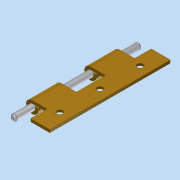
# Autodesk Inventor part: DIV
Saved by Autodesk Inventor 2012 SP1 (Build 160190100, 190)
## iProperties
Created: 2014-07-01
Material: Ms58
Document SubType Name: Modeling
Designer: Eisele
Density: 8.47 g/cm^3
Description: Schanier
Mass: 17.612 g
Surface Area: 32.73 cm^2
Volume: 2.07934 cm^3
Benennung: Schanier
Unterbennenung: 30x26x0,9
Projekt: DIV
Unterprojekt: Schanier
Author: Eisele
Title: DIV
Autodesk Inventor part; units mm, degrees
ref_plane "YZ Plane" through (0, 0, 0) normal (1, 0, 0) x (0, 1, 0)
ref_plane "XZ Plane" through (0, 0, 0) normal (0, 1, 0) x (-1, 0, 0)
ref_plane "XY Plane" through (0, 0, 0) normal (0, 0, 1) x (1, 0, 0)
sketch "Skizze1" plane through (0, 0, 0) normal (0, 1, 0) x (-1, 0, 0)
  line L0 (0, 0) -> (0, 79.9753) construction
  line L1 (0, 0) -> (-80.4332, 0) construction
  line L2 (0, 0) -> (80.1339, 0) construction
  line L3 (0, 0) -> (0, -79.3949) construction
  line L4 (0, 1.55) -> (-17, 1.55)
  line L5 (-17, 1.55) -> (-17, 2.95)
  line L6 (-17, 2.95) -> (0, 2.95)
  arc A0 (-1.3565, 0.75) -> (0, 1.55) centre (0, 0) ccw
  arc A1 (-2.8531, 0.75) -> (0, 2.95) centre (0, 0) ccw
  line L7 (-1.3565, 0.75) -> (-2.8531, 0.75)
  circle A2 centre (0, 0) radius 1.5
  dimension "d0" = 1.4
  dimension "d1" = 5.9
  dimension "d2" = 0.8
  dimension "d3" = 19.95
  dimension "d21" = 0.05
  dimension "d27" = 17
  constraints: 16 end point, 4 perpendicular, 4 point on circle, 3 centre point, 3 coincident, 2 parallel, 2 tangent, 1 collinear, 1 vertical
  measures "d0" distance between parallel lines of L6 L4
  measures "d1" diameter of A1
  measures "d2" distance between parallel lines of L4 L7
  measures "d21" radial gap between concentric circles of A0 A2
  measures "d27" distance from line of L4.end L3
extrude "Extrusion1" add sketch "Skizze1" along normal mid plane 60 contours L4 L5 L6 A1 L7 A0
sketch "Skizze3" plane through (0, 0, 0) normal (0, 0, 1) x (1, 0, 0)
  line L0 (5, -7.25) -> (-9.5, -7.25)
  line L1 (-9.5, -7.25) -> (-9.5, 7.25)
  line L2 (-9.5, 7.25) -> (5, 7.25)
  line L3 (5, 7.25) -> (5, -7.25)
  line L4 (17, 30) -> (17, -30) construction
  line L5 (-11.8, 0) -> (21.8, 0) construction
  point P0 (0, 0)
  dimension "d6" = 12
  dimension "d7" = 14.5
  dimension "d8" = 7.25
  dimension "d9" = 14.5
  constraints: 8 end point, 2 parallel, 1 horizontal, 1 perpendicular
  measures "d6" distance between parallel lines of L4 L3
  measures "d7" distance of L0.end L1.end
  measures "d8" distance between parallel lines of L5 L2
  measures "d9" distance of L1.end L2.end
extrude "Extrusion2" cut sketch "Skizze3" along normal through all both and the other way through all
sketch "Skizze4" plane through (17, 30, 1.55) normal (0, 0, -1) x (-1, 0, 0)
  line L0 (17, -72) -> (17, 12) projected
  line L1 (-3.99, -30) -> (23.94, -30) construction
  line L2 (5, -7.5) -> (5, -52.5) construction
  line L3 (0, 0) -> (0, -60) construction
  point P0 (17, -30)
  point P1 (5, -30)
  dimension "d12" = 45
  dimension "d13" = 5
  constraints: 2 coincident, 2 end point, 1 midpoint, 1 perpendicular, 1 symmetric about line
  measures "d12" distance of L2.start L2.end
  measures "d13" distance between parallel lines of L2 L3
hole "Bohrung1" at (12, 22.5, 1.55) at (12, -22.5, 1.55) at (12, 0, 1.55) direction (0, 0, 1) diameter 3 end through all countersink diameter 4 countersink angle 90
extrude "Extrusion3" add sketch "Skizze1" along normal mid plane 63 separate body contours A2
chamfer "Fase1" distance 0.8 angle 45 2 edges at (1.5, 31.5, 0) (1.5, -31.5, 0)
pattern_linear "Rechteckige Anordnung1" count 3 spacing 29 along (0, 1, 0) of "Extrusion2" first direction both ways yes bodies 1
equation "\"d8\" = 0.5 * d7"
equation "\"d9\" = d7"
